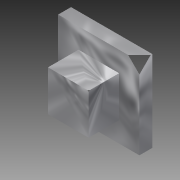
# Autodesk Inventor part: ColdFingerBase
Saved by Autodesk Inventor 2014 (Build 180170000, 170)
## iProperties
Created: 2015-04-18
Part Number: ColdFingerBase
Material: Generic
Document SubType Name: Modeling
Designer: Owner
Density: 1 g/cm^3
Appearance: Aluminum - Polished
Author: Owner
Autodesk Inventor part; units mm, degrees
ref_plane "YZ Plane" through (0, 0, 0) normal (1, 0, 0) x (0, 1, 0)
ref_plane "XZ Plane" through (0, 0, 0) normal (0, 1, 0) x (-1, 0, 0)
ref_plane "XY Plane" through (0, 0, 0) normal (0, 0, 1) x (1, 0, 0)
sketch "Sketch2" plane through (0, 0, 0) normal (0, 0, 1) x (1, 0, 0)
  line L0 (-19.5826, 21.0671) -> (20.4174, 21.0671)
  line L1 (20.4174, 21.0671) -> (20.4174, -18.9329)
  line L2 (20.4174, -18.9329) -> (-19.5826, -18.9329)
  line L3 (-19.5826, -18.9329) -> (-19.5826, 21.0671)
  line L4 (-29.5826, 6.4671) -> (-19.5826, 6.4671)
  line L5 (-19.5826, 6.4671) -> (-19.5826, -18.9329)
  line L6 (-19.5826, -18.9329) -> (-29.5826, -18.9329)
  line L7 (-29.5826, -18.9329) -> (-29.5826, 6.4671)
  line L8 (20.4174, -18.9329) -> (30.4174, -18.9329)
  line L9 (30.4174, -18.9329) -> (30.4174, 6.4671)
  line L10 (30.4174, 6.4671) -> (20.4174, 6.4671)
  line L11 (20.4174, 6.4671) -> (20.4174, -18.9329)
  point P0 (0, 0)
  dimension "d0" = 40
  dimension "d1" = 40
  dimension "d10" = 10
  dimension "d11" = 10
  dimension "d12" = 25.4
  dimension "d13" = 25.4
  constraints: 24 end point, 6 parallel, 3 horizontal, 3 perpendicular
  measures "d0" distance of L0.start L0.end
  measures "d1" distance of L0.end L1.end
  measures "d10" distance of L9.end L10.end
  measures "d11" distance of L4.start L4.end
  measures "d12" distance of L8.end L9.end
  measures "d13" distance of L6.end L4.start
extrude "Extrusion1" add sketch "Sketch2" along normal blind 6.35
sketch "Sketch3" plane through (0, 0, 6.35) normal (0, 0, 1) x (1, 0, 0)
  line L0 (20.4174, 21.0671) -> (-19.5826, 21.0671) projected
  line L1 (20.4174, 6.4671) -> (20.4174, 21.0671) projected
  line L2 (-9.5826, 11.0671) -> (10.4174, 11.0671)
  line L3 (10.4174, 11.0671) -> (10.4174, -8.9329)
  line L4 (10.4174, -8.9329) -> (-9.5826, -8.9329)
  line L5 (-9.5826, -8.9329) -> (-9.5826, 11.0671)
  point P0 (20.4174, -18.9329)
  point P1 (0, 0)
  dimension "d4" = 20
  dimension "d5" = 20
  dimension "d6" = 10
  dimension "d7" = 10
  constraints: 8 end point, 2 parallel, 1 horizontal, 1 perpendicular
  measures "d4" distance of L2.start L2.end
  measures "d5" distance of L2.end L3.end
  measures "d6" distance between parallel lines of L0 L2
  measures "d7" distance between parallel lines of L1 L3
extrude "Extrusion2" add sketch "Sketch3" along normal blind 13
sketch "Sketch4" plane through (20.4174, 6.4671, 0) normal (1, 0, 0) x (0, 0, -1)
  point P0 (-3.175, -19.05)
hole "Hole1" at (20.4174, -12.5829, 3.175) direction (-1, 0, 0) diameter 2.4867 depth 10.475 tip angle 120 thread size "5-40 UNC" class "2B" standard "ANSI Unified Screw Threads"
body "Solid1"
